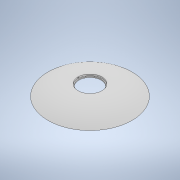
# Autodesk Inventor part: topplock
Saved by Autodesk Inventor 2020 (Build 240168000, 168)
## iProperties
Created: 2020-03-24
Part Number: topplock
Material: Generic
Document SubType Name: Modeling
Designer: magnu
Density: 1 g/cm^3
Appearance: Default
Mass: 97.1698 g
Surface Area: 679.717 cm^2
Volume: 97.1698 cm^3
Author: magnu
Autodesk Inventor part; units mm, degrees
ref_plane "XZ Plane" through (0, 0, 0) normal (0, 1, 0) x (-1, 0, 0)
ref_plane "XY Plane" through (0, 0, 0) normal (0, 0, 1) x (1, 0, 0)
sketch "Sketch1" plane through (0, 0, 0) normal (0, 0, 1) x (1, 0, 0)
  line L0 (0, 30.8148) -> (40, 30.8148)
  line L1 (40, 30.8148) -> (40, 35.8148)
  line L2 (0, 30.8148) -> (0, 0)
  line L3 (0, 0) -> (140, 0)
  arc A0 (140, 0) -> (40, 35.8148) centre (40.5629, -120.1278) ccw
  dimension "d0" = 40
  dimension "d1" = 5
  dimension "d2" = 140
  constraints: 8 end point, 2 perpendicular, 2 point on circle, 1 centre point, 1 horizontal, 1 vertical
  measures "d0" distance of L0.start L0.end
  measures "d1" distance of L0.end L1.end
  measures "d2" distance of L2.end L3.end
revolve "Revolution1" add sketch "Sketch1" angle 360 about axis through (0, 30.8148, 0) along (0, -1, 0)
shell "Shell1" thickness 3 removed faces 1 at (22.2847, 0, -49.1516)
sketch "Sketch2" plane through (0, 30.8148, 0) normal (0, 1, 0) x (1, 0, 0)
  circle A0 centre (0, 0) radius 37
  dimension "d5" = 74
  constraints: 1 centre point, 1 coincident
  measures "d5" diameter of A0
extrude "Extrusion1" cut sketch "Sketch2" against normal through all
ref_plane "Work Plane1" through (40, 33.3148, 0) normal (1, 0, 0) x (0, 1, 0)
sketch "Sketch4" plane through (40, 33.3148, 0) normal (1, 0, 0) x (0, 1, 0)
  line L0 (1, -1.0043) -> (-1, -1.0043)
  line L1 (-1, -1.0043) -> (-1, 0.9957)
  line L2 (-1, 0.9957) -> (1, 0.9957)
  line L3 (1, 0.9957) -> (1, -1.0043)
  line L4 (-2.5, 40) -> (-2.5, -40) projected
  point P0 (-33.3148, 0)
  dimension "d8" = 2
  dimension "d9" = 2
  dimension "d10" = 1.5
  constraints: 8 end point, 2 parallel, 1 horizontal, 1 perpendicular
  measures "d8" distance of L1.end L2.end
  measures "d9" distance of L0.end L1.end
  measures "d10" distance between parallel lines of L4 L1
extrude "Extrusion2" add sketch "Sketch4" against normal blind 2
pattern_circular "Circular Pattern1" count 2 over 360 about axis through (0, 30.8148, 0) along (0, -1, 0) of "Extrusion2"
equation "\"d9\" = d8"
body "Solid1"
